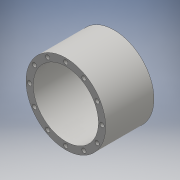
# Autodesk Inventor part: drive_sprocket_middle
Saved by Autodesk Inventor 2016 (Build 200138000, 138)
## iProperties
Created: 2016-11-20
Part Number: drive_sprocket_middle
Material: Generic
Document SubType Name: Modeling
Designer: hesaon
Density: 1 g/cm^3
Appearance: Default
Author: hesaon
Autodesk Inventor part; units mm, degrees
ref_plane "YZ Plane" through (0, 0, 0) normal (1, 0, 0) x (0, 1, 0)
ref_plane "XZ Plane" through (0, 0, 0) normal (0, 1, 0) x (-1, 0, 0)
ref_plane "XY Plane" through (0, 0, 0) normal (0, 0, 1) x (1, 0, 0)
sketch "Sketch1" plane through (0, 0, 0) normal (0, 1, 0) x (-1, 0, 0)
  circle A0 centre (0, 0) radius 18
  circle A1 centre (0, 0) radius 22
  dimension "d0" = 36
  dimension "d1" = 44
  constraints: 2 centre point, 2 coincident
  measures "d0" diameter of A0
  measures "d1" diameter of A1
extrude "Extrusion1" add sketch "Sketch1" along normal blind 26.68
sketch "Sketch2" plane through (0, 26.68, 0) normal (0, 1, 0) x (1, 0, 0)
  circle A0 centre (-20, 0) radius 1.175
  circle A1 centre (-17.3205, -10) radius 1.175
  circle A2 centre (-10, -17.3205) radius 1.175
  circle A3 centre (0, -20) radius 1.175
  circle A4 centre (10, -17.3205) radius 1.175
  circle A5 centre (17.3205, -10) radius 1.175
  circle A6 centre (20, 0) radius 1.175
  circle A7 centre (17.3205, 10) radius 1.175
  circle A8 centre (10, 17.3205) radius 1.175
  circle A9 centre (0, 20) radius 1.175
  circle A10 centre (-10, 17.3205) radius 1.175
  circle A11 centre (-17.3205, 10) radius 1.175
  point P0 (0, 0)
  dimension "d4" = 2.35
  dimension "d5" = 0
  dimension "d6" = 20
  dimension "d9" = 360
  constraints: 12 centre point, 25 other
  measures "d4" diameter of A0
  measures "d5" vertical distance of point (0, 0) A0.centre
  measures "d6" distance of point (0, 0) A0.centre
extrude "Extrusion2" cut sketch "Sketch2" against normal through all
body "Solid1"
